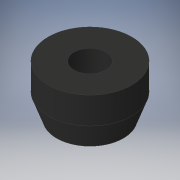
# Autodesk Inventor part: BushingBottom
Saved by Autodesk Inventor 2019 (Build 230136000, 136)
## iProperties
Created: 2020-12-10
Part Number: BushingBottom
Material: Rubber, Black
Document SubType Name: Modeling
Designer: Anass Hamdi
Density: 0.93 g/cm^3
Appearance: Rubber - Black
Author: Anass Hamdi
Autodesk Inventor part; units mm, degrees
ref_plane "YZ Plane" through (0, 0, 0) normal (1, 0, 0) x (0, 1, 0)
ref_plane "XZ Plane" through (0, 0, 0) normal (0, 1, 0) x (-1, 0, 0)
ref_plane "XY Plane" through (0, 0, 0) normal (0, 0, 1) x (1, 0, 0)
sketch "Sketch1" plane through (0, 0, 0) normal (0, 0, 1) x (1, 0, 0)
  line L0 (0, 0) -> (0, 7) construction
  line L1 (0, 7) -> (-20.6567, 7) construction
  line L2 (0, 7) -> (0, 15) construction
  line L3 (-12.5, 15) -> (-12.5, 7)
  line L4 (-12.5, 7) -> (-10, 0)
  line L5 (-12.5, 15) -> (-4.7, 15)
  line L6 (-4.7, 15) -> (-4.7, 0)
  line L7 (-4.7, 0) -> (-10, 0)
  dimension "d0" = 10
  dimension "d1" = 7
  dimension "d2" = 8
  dimension "d3" = 12.5
  dimension "d5" = 4.7
  constraints: 16 end point, 3 perpendicular, 2 horizontal, 2 vertical, 1 point on line
  measures "d0" distance of L0.start L4.end
  measures "d1" distance of L0.start L0.end
  measures "d2" distance of L0.end L2.end
  measures "d3" distance of L2.end L3.start
  measures "d5" distance of L2.end L5.end
revolve "Revolution1" add sketch "Sketch1" angle 360 about axis through (0, 7, 0) along (0, 1, 0)
body "Solid1"
